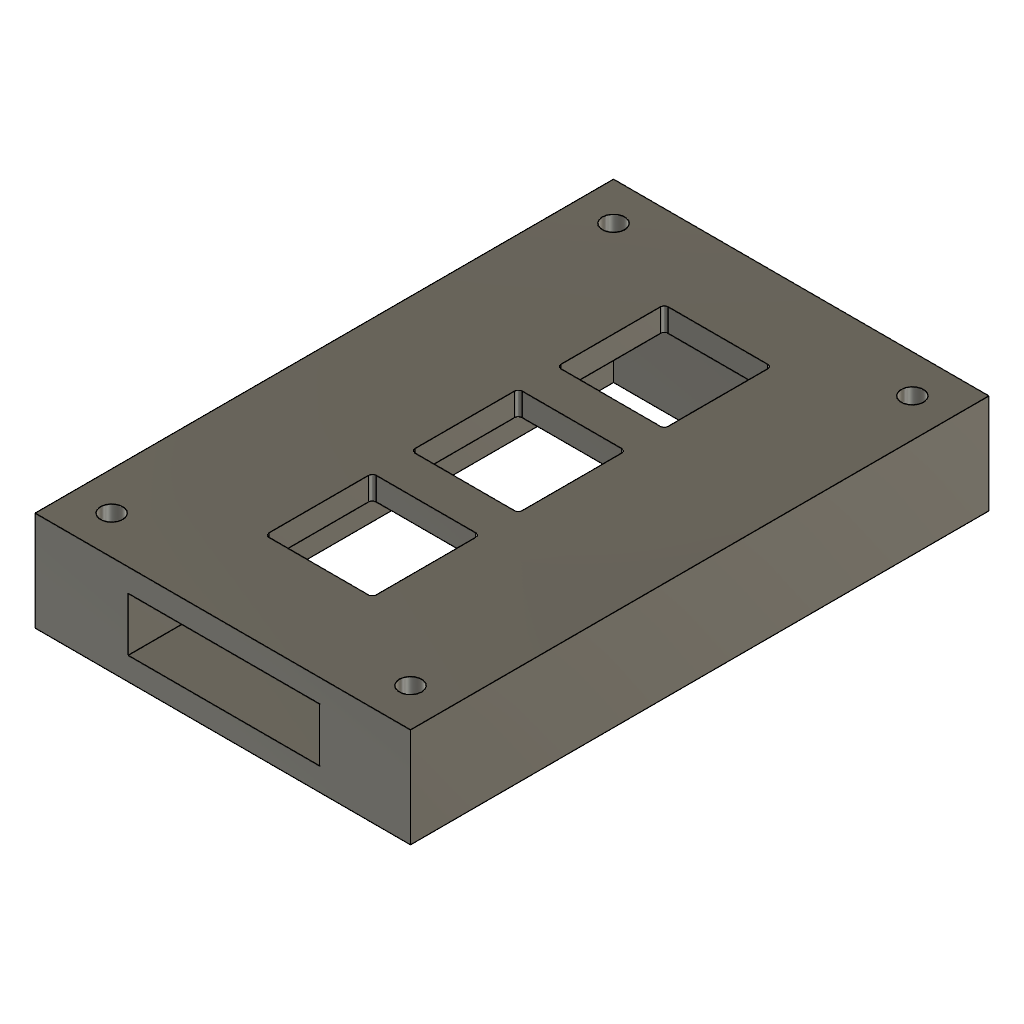
HackPad (Autodesk Fusion 360 design; units mm, degrees)
Autodesk Fusion 360 part; units mm, degrees
sketch "Sketch1" plane through (0, 0, 0) normal (0, 0, 1) x (1, 0, 0)
  line L0 (12.8502, 36.2265) -> (41.8502, 36.2265)
  line L1 (41.8502, 36.2265) -> (41.8502, -19.2735)
  line L2 (41.8502, -19.2735) -> (12.8502, -19.2735)
  line L3 (12.8502, -19.2735) -> (12.8502, 36.2265)
  line L4 (51.8502, 46.2265) -> (51.8502, -29.2735)
  line L5 (51.8502, -29.2735) -> (2.8502, -29.2735)
  line L6 (2.8502, -29.2735) -> (2.8502, 46.2265)
  line L7 (2.8502, 46.2265) -> (51.8502, 46.2265)
  line L8 (51.8502, -29.2735) -> (46.8502, -29.2735)
  line L9 (46.8502, -29.2735) -> (46.8502, 46.2265)
  line L10 (51.8502, -29.2735) -> (51.8502, -24.2735)
  line L11 (51.8502, -24.2735) -> (2.8502, -24.2735)
  line L12 (2.8502, -29.2735) -> (7.8502, -29.2735)
  line L13 (7.8502, -29.2735) -> (7.8502, 46.2265)
  line L14 (2.8502, 46.2265) -> (2.8502, 41.2265)
  line L15 (2.8502, 41.2265) -> (51.8502, 41.2265)
  circle A0 centre (46.8502, -24.2735) radius 1.45
  circle A1 centre (7.8502, -24.2735) radius 1.45
  circle A2 centre (46.8502, 41.2265) radius 1.45
  circle A3 centre (7.8502, 41.2265) radius 1.45
  line L16 (41.8502, -19.2735) -> (27.3502, -19.2735)
  line L17 (36.8752, -19.2735) -> (36.8752, 37.8765)
  line L18 (34.3502, 2.8015) -> (34.3502, 15.8015)
  line L19 (20.3502, 2.8015) -> (20.3502, 15.8015)
  line L20 (17.8252, -19.2735) -> (17.8252, 37.8765)
  line L21 (17.8252, -19.2735) -> (17.8252, 37.8765)
  line L22 (34.3502, 2.8015) -> (34.3502, 15.8015)
  line L23 (20.3502, 2.8015) -> (20.3502, 15.8015)
  line L24 (34.3502, -16.2485) -> (34.3502, -3.2485)
  arc A4 (20.3502, 2.8015) -> (20.8502, 2.3015) centre (20.8502, 2.8015) ccw
  arc A5 (34.3502, 34.8515) -> (33.8502, 35.3515) centre (33.8502, 34.8515) ccw
  line L25 (36.8752, -19.2735) -> (36.8752, 37.8765)
  arc A6 (20.3502, -16.2485) -> (20.8502, -16.7485) centre (20.8502, -16.2485) ccw
  arc A7 (33.8502, -16.7485) -> (34.3502, -16.2485) centre (33.8502, -16.2485) ccw
  line L26 (20.8502, -2.7485) -> (33.8502, -2.7485)
  line L27 (36.8752, -19.2735) -> (17.8252, -19.2735)
  line L28 (20.8502, 21.3515) -> (33.8502, 21.3515)
  arc A8 (33.8502, -16.7485) -> (34.3502, -16.2485) centre (33.8502, -16.2485) ccw
  line L29 (34.3502, -16.2485) -> (34.3502, -3.2485)
  line L30 (20.8502, 35.3515) -> (33.8502, 35.3515)
  line L31 (36.8752, 37.8765) -> (17.8252, 37.8765)
  line L32 (20.8502, 35.3515) -> (33.8502, 35.3515)
  arc A9 (20.8502, -2.7485) -> (20.3502, -3.2485) centre (20.8502, -3.2485) ccw
  line L33 (20.8502, 2.3015) -> (33.8502, 2.3015)
  arc A10 (20.3502, 21.8515) -> (20.8502, 21.3515) centre (20.8502, 21.8515) ccw
  arc A11 (33.8502, 2.3015) -> (34.3502, 2.8015) centre (33.8502, 2.8015) ccw
  arc A12 (20.8502, -2.7485) -> (20.3502, -3.2485) centre (20.8502, -3.2485) ccw
  line L34 (20.3502, -16.2485) -> (20.3502, -3.2485)
  line L35 (20.8502, -2.7485) -> (33.8502, -2.7485)
  arc A13 (34.3502, -3.2485) -> (33.8502, -2.7485) centre (33.8502, -3.2485) ccw
  line L36 (20.3502, 21.8515) -> (20.3502, 34.8515)
  arc A14 (34.3502, 34.8515) -> (33.8502, 35.3515) centre (33.8502, 34.8515) ccw
  arc A15 (20.3502, 21.8515) -> (20.8502, 21.3515) centre (20.8502, 21.8515) ccw
  arc A16 (20.3502, -16.2485) -> (20.8502, -16.7485) centre (20.8502, -16.2485) ccw
  line L37 (36.8752, -19.2735) -> (17.8252, -19.2735)
  line L38 (36.8752, 37.8765) -> (17.8252, 37.8765)
  arc A17 (20.3502, 2.8015) -> (20.8502, 2.3015) centre (20.8502, 2.8015) ccw
  line L39 (20.3502, -16.2485) -> (20.3502, -3.2485)
  arc A18 (34.3502, -3.2485) -> (33.8502, -2.7485) centre (33.8502, -3.2485) ccw
  arc A19 (34.3502, 15.8015) -> (33.8502, 16.3015) centre (33.8502, 15.8015) ccw
  arc A20 (20.8502, 35.3515) -> (20.3502, 34.8515) centre (20.8502, 34.8515) ccw
  arc A21 (34.3502, 15.8015) -> (33.8502, 16.3015) centre (33.8502, 15.8015) ccw
  line L40 (34.3502, 21.8515) -> (34.3502, 34.8515)
  line L41 (20.8502, -16.7485) -> (33.8502, -16.7485)
  line L42 (20.8502, 21.3515) -> (33.8502, 21.3515)
  line L43 (20.3502, 21.8515) -> (20.3502, 34.8515)
  line L44 (20.8502, 2.3015) -> (33.8502, 2.3015)
  line L45 (34.3502, 21.8515) -> (34.3502, 34.8515)
  arc A22 (33.8502, 2.3015) -> (34.3502, 2.8015) centre (33.8502, 2.8015) ccw
  arc A23 (20.8502, 35.3515) -> (20.3502, 34.8515) centre (20.8502, 34.8515) ccw
  line L46 (20.8502, -16.7485) -> (33.8502, -16.7485)
  arc A24 (20.8502, 16.3015) -> (20.3502, 15.8015) centre (20.8502, 15.8015) ccw
  arc A25 (33.8502, 21.3515) -> (34.3502, 21.8515) centre (33.8502, 21.8515) ccw
  line L47 (20.8502, 16.3015) -> (33.8502, 16.3015)
  arc A26 (33.8502, 21.3515) -> (34.3502, 21.8515) centre (33.8502, 21.8515) ccw
  arc A27 (20.8502, 16.3015) -> (20.3502, 15.8015) centre (20.8502, 15.8015) ccw
  line L48 (20.8502, 16.3015) -> (33.8502, 16.3015)
  line L49 (36.8752, -19.2735) -> (28.3002, -19.2735)
  line L50 (36.8752, -19.2735) -> (27.3502, -19.2735)
  dimension "d1" = 29
  dimension "d2" = 55.5
  dimension "d3" = -10
  dimension "d4" = 5
  dimension "d5" = 5
  dimension "d6" = 5
  dimension "d7" = 5
  dimension "d8" = 2.9
  dimension "d9" = 2.9
  dimension "d10" = 2.9
  dimension "d11" = 2.9
  constraint horizontal L0
  constraint vertical L1
  constraint horizontal L2
  constraint vertical L3
  constraint perpendicular L4 L8
  constraint coincident L7 L9.end
  constraint perpendicular L7 L9
  constraint perpendicular L8 L10
  constraint coincident L6 L11.end
  constraint perpendicular L6 L11
  constraint perpendicular L6 L12
  constraint coincident L7 L13.end
  constraint perpendicular L7 L13
  constraint perpendicular L7 L14
  constraint coincident L4 L15.end
  constraint perpendicular L4 L15
  constraint coincident L11 A0.centre
  constraint coincident L9 A0.centre
  constraint coincident L13 A1.centre
  constraint coincident L11 A1.centre
  constraint coincident L15 A2.centre
  constraint coincident L9 A2.centre
  constraint coincident L13 A3.centre
  constraint coincident L15 A3.centre
  constraint midpoint L2 L16.end
  constraint coincident L37 L49.end
  constraint perpendicular L17 L49
  constraint midpoint L37 L16.end
  constraint perpendicular L17 L50
  measures "d1" distance of L0.start L0.end
  measures "d2" distance of L0.start L2.end
  measures "d4" distance of L4.end L8.end
  measures "d5" distance of L4.end L10.end
  measures "d6" distance of L5.end L12.end
  measures "d7" distance of L6.end L14.end
  measures "d8" diameter of A0
  measures "d9" diameter of A1
  measures "d10" diameter of A2
  measures "d11" diameter of A3
extrude "Extrude1" add sketch "Sketch1" along normal blind 3 contours L0 L2 L3 L20 L21 | L0 L17 L20 L21 L25 L31 L38 | L0 L2 L16 L17 L20 L21 L25 L27 L37 L49 L50 | L0 L1 L2 L16 L17 L25 | L4 L7 L9 L15 A2 | L4 L9 L11 L15 A0 A2 | L7 L9 L13 L15 A2 A3 | L4 L5 L8 L9 L10 L11 A0 | L6 L7 L13 L14 L15 A3 | L9 L11 L13 L15 A0 A1 A2 A3 | L5 L9 L11 L13 A0 A1 | L6 L11 L13 L15 A1 A3 | L5 L6 L11 L12 L13 A1 | L18 L19 L22 L23 A4 L33 A11 A17 A19 A21 L44 A22 A24 L47 A27 L48 | L24 A6 A7 L26 A8 L29 A9 A12 L34 L35 A13 A16 L39 A18 L41 L46 | A5 L28 L30 L32 A10 L36 A14 A15 A20 L40 L42 L43 L45 A23 A25 A26
extrude "Extrude2" add sketch "Sketch1" against normal blind 10 contours L0 L17 L20 L21 L25 L31 L38 | L4 L7 L9 L15 A2 | L4 L9 L11 L15 A0 A2 | L7 L9 L13 L15 A2 A3 | L4 L5 L8 L9 L10 L11 A0 | L6 L7 L13 L14 L15 A3 | L9 L11 L13 L15 A0 A1 A2 A3 | L5 L9 L11 L13 A0 A1 | L6 L11 L13 L15 A1 A3 | L5 L6 L11 L12 L13 A1
extrude "Extrude3" cut sketch "Sketch1" along normal blind 10 contours L18 L19 L22 L23 A4 L33 A11 A17 A19 A21 L44 A22 A24 L47 A27 L48 | L24 A6 A7 L26 A8 L29 A9 A12 L34 L35 A13 A16 L39 A18 L41 L46 | A5 L28 L30 L32 A10 L36 A14 A15 A20 L40 L42 L43 L45 A23 A25 A26
sketch "Sketch3" plane through (0, -29.2735, 0) normal (0, -1, 0) x (1, 0, 0)
  line L0 (51.8502, -10) -> (51.8502, 3)
  line L1 (51.8502, 3) -> (2.8502, 3)
  line L2 (2.8502, 3) -> (2.8502, -10)
  line L3 (2.8502, -10) -> (51.8502, -10)
  line L4 (40, 0) -> (15, 0)
  line L5 (15, 0) -> (15, -7)
  line L6 (15, -7) -> (40, -7)
  line L7 (40, -7) -> (40, 0)
  constraint horizontal L4
  constraint vertical L5
  constraint horizontal L6
  constraint vertical L7
extrude "Extrude4" cut sketch "Sketch3" against normal blind 19 contours L4 L5 L6 L7
